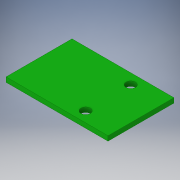
# Autodesk Inventor part: temp_probe_board
Saved by Autodesk Inventor 2017 (Build 210142000, 142)
## iProperties
Created: 2017-07-30
Part Number: temp_probe_board
Material: Generic
Document SubType Name: Modeling
Designer: Mitch
Density: 1 g/cm^3
Appearance: Dark Green
Author: Mitch
Autodesk Inventor part; units mm, degrees
ref_plane "YZ Plane" through (0, 0, 0) normal (1, 0, 0) x (0, 1, 0)
ref_plane "XZ Plane" through (0, 0, 0) normal (0, 1, 0) x (-1, 0, 0)
ref_plane "XY Plane" through (0, 0, 0) normal (0, 0, 1) x (1, 0, 0)
sketch "Sketch1" plane through (0, 0, 0) normal (0, 1, 0) x (-1, 0, 0)
  line L0 (0, 0) -> (34.163, 0)
  line L1 (34.163, 0) -> (34.163, -22.098)
  line L2 (34.163, -22.098) -> (0, -22.098)
  line L3 (0, -22.098) -> (0, 0)
  dimension "d0" = 34.163
  dimension "d1" = 22.098
  constraints: 8 end point, 2 parallel, 1 horizontal, 1 perpendicular
  measures "d0" distance of L1.end L2.end
  measures "d1" distance of L0.end L1.end
extrude "Extrusion1" add sketch "Sketch1" along normal blind 1.5748
hole "Hole2" at (-10.9855, 1.5748, -3.4925) direction (0, -1, 0) diameter 3.175 depth 25.4 tip angle 118
hole "Hole3" at (-10.9855, 1.5748, -18.6055) direction (0, -1, 0) diameter 3.175 depth 25.4 tip angle 118
body "Solid1"
